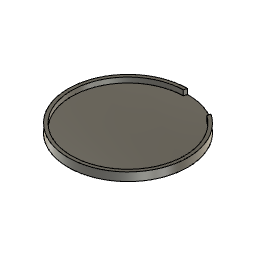
respeaker stand v1 (Autodesk Fusion 360 design; units mm, degrees)
Autodesk Fusion 360 part; units mm, degrees
note: some values were not read from the file. Set by a fixed rule: which sketch regions a step uses.
sketch "Sketch1" plane through (0, 0, 0) normal (0, 0, 1) x (1, 0, 0)
  circle A0 centre (0, 0) radius 37
  dimension "d1" = 74
  constraint coincident A0.centre origin
  measures "d1" diameter of A0
extrude "Extrude1" add sketch "Sketch1" along normal blind 3.2
shell "Shell1" thickness 2 removed faces 1 at (-10.1246, 15.5782, 3.2)
sketch "Sketch2" plane through (0, 0, 3.2) normal (0, 0, 1) x (-1, 0, 0)
  circle A0 centre (0, 0) radius 35
  circle A1 centre (0, 0) radius 37
  line L0 (0.7607, -34.9917) -> (-20.2884, -28.5935)
  line L1 (-20.2884, -28.5935) -> (-21.7759, -33.4571)
  line L2 (-21.7759, -33.4571) -> (-0.7372, -39.8892)
  line L3 (-0.7372, -39.8892) -> (0.7607, -34.9917)
  dimension "d5" = 22
  constraint coincident A0 L0.start
  measures "d5" distance of L0.start L0.end
extrude "Extrude2" cut sketch "Sketch2" against normal blind 1.2 contours A0 A1 L0 L1 L3 picked at (-0.9203, -35.5996)
extrude "Extrude3" add 1 faces at (35.2522, 4.9796, 3.2) along direction (0, 0, 1) blind 2
